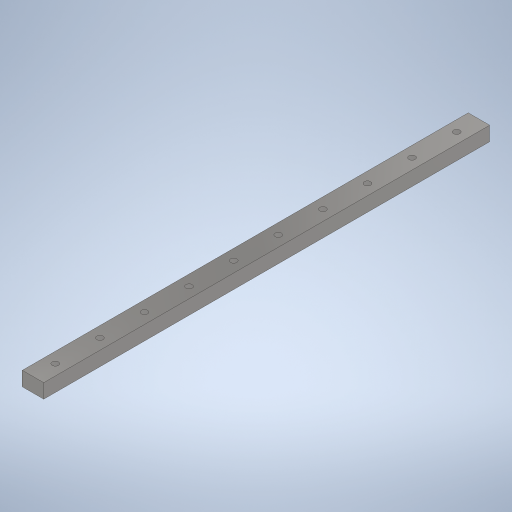
# Autodesk Inventor part: MGN12H_rail
Saved by Autodesk Inventor 2024 (Build 280153000, 153)
## iProperties
Created: 2023-08-27
Part Number: MGN12H_rail
Material: Stainless Steel
Document SubType Name: Modeling
Designer: l1534
Density: 8 g/cm^3
Appearance: Semi-Polished
Author: l1534
Autodesk Inventor part; units mm, degrees
ref_plane "YZ Plane" through (0, 0, 0) normal (1, 0, 0) x (0, 1, 0)
ref_plane "XZ Plane" through (0, 0, 0) normal (0, 1, 0) x (-1, 0, 0)
ref_plane "XY Plane" through (0, 0, 0) normal (0, 0, 1) x (1, 0, 0)
sketch "Sketch1" plane through (0, 0, 0) normal (0, 1, 0) x (-1, 0, 0)
  line L0 (-47.4268, -17.2867) -> (-59.4268, -17.2867)
  line L1 (-59.4268, -17.2867) -> (-59.4268, 232.7133)
  line L2 (-59.4268, 232.7133) -> (-47.4268, 232.7133)
  line L3 (-47.4268, 232.7133) -> (-47.4268, -17.2867)
  point P0 (0, 0)
  dimension "d0" = 250
  dimension "d1" = 12
  constraints: 8 end point, 2 parallel, 1 horizontal, 1 perpendicular
  measures "d0" distance of L0.end L1.end
  measures "d1" distance of L0.start L0.end
extrude "Extrusion1" add sketch "Sketch1" along normal blind 8
sketch "Sketch2" plane through (0, 8, 0) normal (0, 1, 0) x (1, 0, 0)
  circle A0 centre (53.4268, -220.2133) radius 1.75
  line L0 (59.4268, -232.7133) -> (59.4268, 17.2867) projected
  line L1 (47.4268, -232.7133) -> (59.4268, -232.7133) projected
  circle A1 centre (53.4268, -195.2133) radius 1.75
  circle A2 centre (53.4268, -170.2133) radius 1.75
  circle A3 centre (53.4268, -145.2133) radius 1.75
  circle A4 centre (53.4268, -120.2133) radius 1.75
  circle A5 centre (53.4268, -95.2133) radius 1.75
  circle A6 centre (53.4268, -70.2133) radius 1.75
  circle A7 centre (53.4268, -45.2133) radius 1.75
  circle A8 centre (53.4268, -20.2133) radius 1.75
  circle A9 centre (53.4268, 4.7867) radius 1.75
  point P0 (0, 0)
  dimension "d4" = 3.5
  dimension "d5" = 6
  dimension "d6" = 12.5
  dimension "d9" = 25
  constraints: 10 centre point, 1 vertical, 18 other
  measures "d4" diameter of A0
  measures "d5" distance from line of L0 A0.centre
  measures "d6" distance from line of L1 A0.centre
  measures "d9" distance of A0.centre A1.centre
extrude "Extrusion2" cut sketch "Sketch2" against normal through all
body "Solid1"
